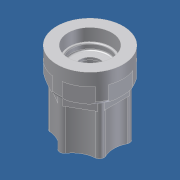
# Autodesk Inventor part: TUB13612
Saved by Autodesk Inventor 2012 SP1 (Build 160190100, 190)
## iProperties
Category: PARTsolutions
Created: 2012-06-06
Part Number: TUB13612
Catalog Web Link: www.cadenas.de
Description: HFC12 End - End
Document SubType Name: Modeling
Designer: PARTsolutions
Material: Default
Mass: 7.74462 g
Surface Area: 52.0622 cm^2
Volume: 7.74462 cm^3
Density: 1 g/cm^3
NB: TUB13612
NN: HFC12 End
NT: End
NBSYN: TUB$PN.
LINA: TUB13612
TS: 3/8" OD
PN: 13612
KT: DUMMY
SUPPLIER: Colder
ARTICLENO: TUB13612HI
BOMINFO: TUB13612
CREATOR: CADENAS GmbH
PSOL_IDENT_0: {\\10.0.0.251\data_v9\23d-libs\colder\single_line\3_8_nom_flow\hfc12_series\bodies\parts\hfc12_hosba
PSOL_IDENT_1: rb_comp.prj},161 {VTYP=3D},{NB=TUB13612},{LINA=TUB13612},{NN=HFC12 End},{DATE=07.08.2007 12:58:33},{
PSOL_IDENT_2: GEOMDATE=07.08.2007 11:22:00},{VERSION=},{LINEID=50},{LINESUBID=-1},{WBVAR=}  {NB=TUB13612},{LINA=TU
PSOL_IDENT_3: B13612},{KT=DUMMY},{TS=3/8\" OD},{PN=13612}
Title: TUB13612
Author: Cadenas PARTsolutions
Comments: End
Autodesk Inventor part; units mm, degrees
sketch "Sketch1" plane through (0, 0, 0) normal (0.5, 0.8660254, 0) x (-0.8660254, 0.5, 0)
  line L0 (0, 0) -> (0, -29.6215)
  arc A0 (-12.7, -9.906) -> (-11.6307, -11.16) centre (-11.43, -9.906) ccw
  line L1 (-11.6307, -11.16) -> (-11.6307, -29.718)
  line L2 (-11.6307, -29.718) -> (-4.826, -29.718)
  line L3 (-4.826, -29.718) -> (-5.9805, -26.8605)
  line L4 (-5.9805, -26.8605) -> (-7.9375, -26.8605)
  line L5 (-7.9375, -26.8605) -> (-7.9375, -26.6831)
  line L6 (-7.9375, -26.6831) -> (-7.3214, -26.3274)
  line L7 (-7.3214, -26.3274) -> (-7.3215, -26.2083)
  line L8 (-7.3215, -26.2083) -> (-7.9375, -25.8527)
  line L9 (-7.9375, -25.8527) -> (-7.9376, -25.4131)
  line L10 (-7.9376, -25.4131) -> (-7.3215, -25.0574)
  line L11 (-7.3215, -25.0574) -> (-7.3214, -24.9383)
  line L12 (-7.3214, -24.9383) -> (-7.9374, -24.5826)
  line L13 (-7.9374, -24.5826) -> (-7.9374, -24.143)
  line L14 (-7.9374, -24.143) -> (-7.3214, -23.7874)
  line L15 (-7.3214, -23.7874) -> (-7.3214, -23.6683)
  line L16 (-7.3214, -23.6683) -> (-7.9375, -23.3126)
  line L17 (-7.9375, -23.3126) -> (-7.9374, -22.873)
  line L18 (-7.9374, -22.873) -> (-7.3214, -22.5174)
  line L19 (-7.3214, -22.5174) -> (-7.3214, -22.3983)
  line L20 (-7.3214, -22.3983) -> (-7.9374, -22.0426)
  line L21 (-7.9374, -22.0426) -> (-7.1374, -22.098)
  line L22 (-7.1374, -22.098) -> (-7.1374, -22.606)
  line L23 (-7.1374, -22.606) -> (-5.9055, -22.606)
  line L24 (-5.9055, -22.606) -> (-4.826, -17.0525)
  line L25 (-4.826, -17.0525) -> (-4.826, -7.747)
  arc A1 (-4.699, -7.62) -> (-4.826, -7.747) centre (-4.699, -7.747) ccw
  line L26 (-4.699, -7.62) -> (-3.9624, -7.62)
  line L27 (-3.9624, -7.62) -> (-3.9624, -6.731)
  line L28 (-3.9624, -6.731) -> (-6.6675, -6.731)
  arc A2 (-7.1755, -6.223) -> (-6.6675, -6.731) centre (-6.6675, -6.223) ccw
  line L29 (-7.1755, -6.223) -> (-7.1755, -4.699)
  arc A3 (-7.1755, -4.699) -> (-7.5565, -4.318) centre (-7.5565, -4.699) ccw
  line L30 (-7.5565, -4.318) -> (-7.7724, -4.318)
  arc A4 (-7.7724, -4.318) -> (-8.1534, -4.699) centre (-7.7724, -4.699) ccw
  line L31 (-8.1534, -4.699) -> (-8.1534, -7.62)
  arc A5 (-8.6614, -8.128) -> (-8.1534, -7.62) centre (-8.6614, -7.62) ccw
  line L32 (-8.6614, -8.128) -> (-9.0297, -8.128)
  arc A6 (-9.7917, -7.366) -> (-9.0297, -8.128) centre (-9.0297, -7.366) ccw
  line L33 (-9.7917, -7.366) -> (-9.7917, -5.1873)
  line L34 (-9.7917, -5.1873) -> (-8.763, -6.096)
  line L35 (-8.763, -6.096) -> (-8.382, -6.096)
  line L36 (-8.382, -6.096) -> (-8.382, 0)
  line L37 (-8.382, 0) -> (-12.7, 0)
  line L38 (-12.7, 0) -> (-12.7, -9.906)
  constraints: 78 end point, 14 point on circle, 7 centre point
revolve "Revolution1" add sketch "Sketch1" angle 360 about axis through (0, 0, 0) along (0, 0, 1)
sketch "Sketch4" plane through (0, 0, -4.826) normal (0, 0, -1) x (-1, 0, 0)
  line L0 (-34.7607, 33.7672) -> (-34.7607, -35.0136)
  line L1 (-34.7607, -35.0136) -> (34.6047, -35.0136)
  line L2 (34.6047, -35.0136) -> (34.6047, 33.7672)
  line L3 (34.6047, 33.7672) -> (-34.7607, 33.7672)
  line L4 (-11.811, 6.8191) -> (-11.811, -6.8191)
  line L5 (-11.811, -6.8191) -> (0, -13.6382)
  line L6 (0, -13.6382) -> (11.811, -6.8191)
  line L7 (11.811, -6.8191) -> (11.811, 6.8191)
  line L8 (11.811, 6.8191) -> (0, 13.6382)
  line L9 (0, 13.6382) -> (-11.811, 6.8191)
  constraints: 20 end point
extrude "Extrusion1" cut sketch "Sketch4" along normal blind 7.2075
sketch "Sketch7" plane through (0, 0, -14.0335) normal (0, 0, -1) x (-1, 0, 0)
  line L0 (-40.2976, 35.6926) -> (-40.2976, -38.6798)
  line L1 (-40.2976, -38.6798) -> (42.7056, -38.6798)
  line L2 (42.7056, -38.6798) -> (42.7056, 35.6926)
  line L3 (42.7056, 35.6926) -> (-40.2976, 35.6926)
  arc A0 (-10.3124, -4.92) -> (-9.4171, -6.4708) centre (-8.5217, -4.92) ccw
  line L4 (-9.4171, -6.4708) -> (-0.8954, -11.3908)
  arc A1 (-0.8954, -11.3908) -> (0.8954, -11.3908) centre (0, -9.84) ccw
  line L5 (0.8954, -11.3908) -> (9.417, -6.4708)
  arc A2 (9.417, -6.4708) -> (10.3124, -4.92) centre (8.5217, -4.92) ccw
  line L6 (10.3124, -4.92) -> (10.3124, 4.92)
  arc A3 (10.3124, 4.92) -> (9.4171, 6.4708) centre (8.5217, 4.92) ccw
  line L7 (9.4171, 6.4708) -> (0.8954, 11.3908)
  arc A4 (0.8954, 11.3908) -> (-0.8954, 11.3908) centre (0, 9.84) ccw
  line L8 (-0.8954, 11.3908) -> (-9.4171, 6.4708)
  arc A5 (-9.4171, 6.4708) -> (-10.3124, 4.92) centre (-8.5217, 4.92) ccw
  line L9 (-10.3124, 4.92) -> (-10.3124, -4.92)
  constraints: 20 end point, 12 point on circle, 6 centre point
extrude "Extrusion2" cut sketch "Sketch7" against normal blind 2.8575
sketch "Sketch10" plane through (0, 0, -29.718) normal (0, 0, -1) x (-1, 0, 0)
  line L0 (-27.6117, 44.2818) -> (-27.6117, -40.5432)
  line L1 (-27.6117, -40.5432) -> (32.3428, -40.5432)
  line L2 (32.3428, -40.5432) -> (32.3428, 44.2818)
  line L3 (32.3428, 44.2818) -> (-27.6117, 44.2818)
  arc A0 (-8.6537, 6.7058) -> (-10.1343, 4.1414) centre (-8.5217, 4.92) ccw
  arc A1 (-10.1343, -4.1414) -> (-10.1343, 4.1414) centre (-18.7118, 0) ccw
  arc A2 (-10.1343, -4.1414) -> (-8.6537, -6.7058) centre (-8.5217, -4.92) ccw
  arc A3 (-1.4806, -10.8473) -> (-8.6537, -6.7058) centre (-9.3559, -16.2049) ccw
  arc A4 (-1.4806, -10.8473) -> (1.4806, -10.8473) centre (0, -9.84) ccw
  arc A5 (8.6537, -6.7058) -> (1.4806, -10.8473) centre (9.3559, -16.2049) ccw
  arc A6 (8.6537, -6.7058) -> (10.1343, -4.1414) centre (8.5217, -4.92) ccw
  arc A7 (10.1343, 4.1414) -> (10.1343, -4.1414) centre (18.7118, 0) ccw
  arc A8 (10.1343, 4.1414) -> (8.6537, 6.7058) centre (8.5217, 4.92) ccw
  arc A9 (1.4806, 10.8473) -> (8.6537, 6.7058) centre (9.3559, 16.2049) ccw
  arc A10 (1.4806, 10.8473) -> (-1.4806, 10.8473) centre (0, 9.84) ccw
  arc A11 (-8.6537, 6.7058) -> (-1.4806, 10.8473) centre (-9.3559, 16.2049) ccw
  constraints: 24 point on circle, 12 centre point, 8 end point
extrude "Extrusion3" cut sketch "Sketch10" against normal blind 15.6845
ref_plane "0_XY" through (0, 0, 0) normal (0, 0, 1) x (1, 0, 0)
ref_plane "0_YZ" through (0, 0, 0) normal (1, 0, 0) x (0, 1, 0)
ref_plane "0_ZX" through (0, 0, 0) normal (0, 1, 0) x (0, 0, 1)
body "Solid1"
